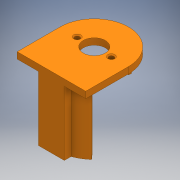
# Autodesk Inventor part: Motor Face Mount
Saved by Autodesk Inventor 2018 (Build 220112000, 112)
## iProperties
Created: 2018-01-11
Part Number: Motor Face Mount
Material: Generic
Document SubType Name: Modeling
Designer: Moochster
Density: 1 g/cm^3
Appearance: Orange
Author: Moochster
Autodesk Inventor part; units mm, degrees
ref_plane "YZ Plane" through (0, 0, 0) normal (1, 0, 0) x (0, 1, 0)
ref_plane "XZ Plane" through (0, 0, 0) normal (0, 1, 0) x (-1, 0, 0)
ref_plane "XY Plane" through (0, 0, 0) normal (0, 0, 1) x (1, 0, 0)
sketch "Sketch1" plane through (0, 0, 0) normal (0, 0, 1) x (1, 0, 0)
  circle A0 centre (0, 0) radius 5.15
  circle A1 centre (0, 0) radius 16
  line L0 (-16, 0) -> (-16, -20)
  line L1 (-16, -20) -> (16, -20)
  line L2 (16, -20) -> (16, 0)
  circle A2 centre (0, 0) radius 14.5
  point P0 (-8, 0)
  point P1 (8, 0)
  dimension "d0" = 10.3
  dimension "d1" = 32
  dimension "d3" = 20
  dimension "d4" = 8
  dimension "d5" = 8
  dimension "d28" = 1.5
  constraints: 6 end point, 3 centre point, 3 coincident, 2 horizontal alignment, 2 perpendicular, 2 point on circle, 2 tangent, 1 vertical
  measures "d0" diameter of A0
  measures "d1" diameter of A1
  measures "d3" distance of L1.end L2.end
  measures "d4" distance of point (0, 0) point (8, 0)
  measures "d5" distance of point (0, 0) point (-8, 0)
  measures "d28" radial gap between concentric circles of A1 A2
extrude "Extrusion1" add sketch "Sketch1" along normal blind 3 contours A1 | L2 L1 L0 A1 | A2
hole "Hole1" at (-8, 0, 0) at (8, 0, 0) direction (0, 0, 1) diameter 2.3 end through all
sketch "Sketch2" plane through (0, 0, 0) normal (0, 0, -1) x (-1, 0, 0)
  arc A0 (1.3828, 14.685) -> (-1.3828, 14.685) centre (0, 0) ccw
  line L0 (-1.3828, 14.685) -> (-1.5, 15.9295)
  arc A1 (16, 0) -> (-16, 0) centre (0, 0) ccw projected
  line L1 (1.3828, 14.685) -> (1.5, 15.9295)
  point P0 (0, 14.75)
  dimension "d15" = 3
  dimension "d16" = 1.25
  constraints: 5 point on circle, 4 end point, 2 line through centre, 1 centre point, 1 concentric, 1 vertical alignment
  measures "d15" distance of L1.end L0.end
  measures "d16" radial gap between concentric circles of A1 A0
extrude "Extrusion2" add sketch "Sketch2" along normal blind 15
sketch "Sketch3" plane through (0, 0, 0) normal (0, 0, -1) x (-1, 0, 0)
  arc A0 (-1.9403, 14.7378) -> (1.9403, 14.7378) centre (0, 0) ccw projected
  arc A1 (-2.3319, 17.7122) -> (2.3319, 17.7122) centre (0, 0) ccw
  line L0 (-6, -16.8273) -> (-6, -20)
  line L1 (-6, -20) -> (6, -20)
  line L2 (16, -20) -> (-16, -20) construction
  line L3 (6, -16.8273) -> (6, -20)
  line L4 (-12, -13.2347) -> (-9.9849, -11.0123)
  line L5 (12, -13.2347) -> (9.9849, -11.0123)
  point P0 (0, 0)
  dimension "d19" = 3
  dimension "d20" = 12
  dimension "d21" = 24
  dimension "d22" = 12
  constraints: 10 end point, 8 point on circle, 2 line through centre, 1 centre point, 1 horizontal, 1 parallel, 1 perpendicular, 1 point on line, 1 vertical
  measures "d19" radial gap between concentric circles of A0 A1
  measures "d20" distance between parallel lines of L0 L3
  measures "d21" distance of L5.start L4.start
  measures "d22" horizontal distance of point (0, 0) L4.start
extrude "Extrusion3" add sketch "Sketch3" along normal blind 30
chamfer "Chamfer1" distance 0.5 angle 45 2 edges at (-8, -1.15, 3) (8, -1.15, 3)
body "Solid1"
